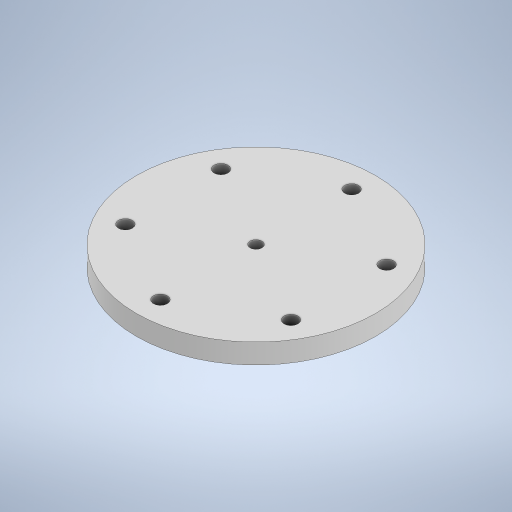
# Autodesk Inventor part: Base
Saved by Autodesk Inventor 2023 (Build 270158000, 158)
## iProperties
Created: 2023-02-08
Part Number: Base
Material: Ogólny
Document SubType Name: Modeling
Designer: kamil
Density: 1 g/cm^3
Appearance: Domyślna
Author: kamil
Autodesk Inventor part; units mm, degrees
ref_plane "YZ Plane" through (0, 0, 0) normal (1, 0, 0) x (0, 1, 0)
ref_plane "XZ Plane" through (0, 0, 0) normal (0, 1, 0) x (-1, 0, 0)
ref_plane "XY Plane" through (0, 0, 0) normal (0, 0, 1) x (1, 0, 0)
sketch "Szkic1" plane through (0, 0, 0) normal (1, 0, 0) x (0, 1, 0)
  line L0 (5, 0) -> (-5, 0)
  line L1 (-5, 0) -> (-5, -19.25)
  line L2 (-5, -60) -> (5, -60)
  line L3 (5, -60) -> (5, 0)
  line L4 (5, 0) -> (5, -32)
  line L5 (5, 0) -> (5, -28.5)
  line L6 (-5, 0) -> (-5, -6)
  line L7 (-7.3, 0) -> (7.05, 0) projected
  line L8 (-5, 0) -> (-5, -33.2566)
  line L9 (-5, 0) -> (-5.25, 0)
  arc A0 (-5, -42.7434) -> (-5, -33.2566) centre (-5.25, -38) ccw
  line L10 (-5, -42.7434) -> (-5, -60)
  line L11 (-5, -28.75) -> (-5, -33.2566)
  line L12 (-5, -42.7434) -> (-5, -60)
  point P0 (0, 0)
  point P1 (0, 0)
  dimension "d0" = 10
  dimension "d1" = 60
  dimension "d44" = 38
  dimension "d48" = 4.75
  constraints: 24 end point, 5 point on line, 4 collinear, 4 parallel, 3 perpendicular, 2 point on circle, 1 centre point, 1 coincident, 1 horizontal, 1 midpoint
  measures "d0" distance of L2.end L2.start
  measures "d1" distance of L2.start L0.end
  measures "d44" vertical distance of L0.end A0.centre
  measures "d48" radius of A0
revolve "Obrót2" add sketch "Szkic1" angle 360 about axis through (0, 5, 0) along (0, -1, 0)
sketch "Szkic4" plane through (0, 5, 0) normal (0, 1, 0) x (1, 0, 0)
  line L0 (0, 0) -> (0, 48)
  circle A0 centre (0, 48) radius 3.5
  circle A1 centre (-41.5692, 24) radius 3.5
  circle A2 centre (-41.5692, -24) radius 3.5
  circle A3 centre (0, -48) radius 3.5
  circle A4 centre (41.5692, -24) radius 3.5
  circle A5 centre (41.5692, 24) radius 3.5
  circle A6 centre (0, 0) radius 3
  dimension "d32" = 48
  dimension "d33" = 7
  dimension "d36" = 360
  dimension "d38" = 6
  constraints: 7 centre point, 4 coincident, 2 end point, 1 vertical, 17 other
  measures "d32" distance of L0.start L0.end
  measures "d33" diameter of A0
  measures "d38" diameter of A6
extrude "Wyciągnięcie proste5" cut sketch "Szkic4" against normal blind 5 contours A0 | A1 | A2 | A3 | A4 | A5
sketch "Szkic5" plane through (0, 5, 0) normal (0, 1, 0) x (1, 0, 0)
  circle A0 centre (0, 0) radius 3
  dimension "d41" = 6
  constraints: 1 centre point, 1 coincident
  measures "d41" diameter of A0
extrude "Wyciągnięcie proste6" cut sketch "Szkic5" against normal blind 10
chamfer "Faza2" distance 0.5 angle 45 2 edges at (0, -5, 42.7434) (0, -5, 33.2566)
